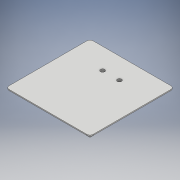
# Autodesk Inventor part: Touchplate
Saved by Autodesk Inventor 2017 (Build 210142000, 142)
## iProperties
Created: 2016-05-03
Part Number: Touchplate
Material: Generic
Document SubType Name: Modeling
Designer: alist
Density: 1 g/cm^3
Appearance: Default
Author: alist
## iProperties of the stored document Touchplate_3DPrint.ipt
Created: 2017-01-15
Part Number: Touchplate_3DPrint
Material: Generic
Document SubType Name: Modeling
Designer: Alistair
Density: 1 g/cm^3
Appearance: Default
Author: Alistair
Autodesk Inventor part; units mm, degrees
ref_plane "YZ Plane" through (0, 0, 0) normal (1, 0, 0) x (0, 1, 0)
ref_plane "XZ Plane" through (0, 0, 0) normal (0, 1, 0) x (-1, 0, 0)
ref_plane "XY Plane" through (0, 0, 0) normal (0, 0, 1) x (1, 0, 0)
sketch "Sketch1" plane through (0, 0, 0) normal (0, 0, 1) x (1, 0, 0)
  circle A0 centre (5, 0) radius 1.1 projected
  circle A1 centre (-11, 0) radius 1.1 projected
  line L0 (-11, 0) -> (5, 0) construction
  line L1 (-43, 20) -> (37, 20)
  line L2 (-3, 22.8039) -> (-3, -25.7358) construction
  line L3 (37, 20) -> (37, -60)
  line L4 (37, -60) -> (-43, -60)
  line L5 (-43, -60) -> (-43, 20)
  point P0 (0, 0)
  point P1 (-3, 0)
  point P2 (-3, 20)
  dimension "d0" = 80
  dimension "d1" = 80
  dimension "d2" = 20
  constraints: 12 end point, 2 horizontal, 2 midpoint, 2 perpendicular, 2 point on line, 2 vertical
  measures "d0" distance of L1.start L1.end
  measures "d1" distance of L1.end L3.end
  measures "d2" distance between parallel lines of L1 L0
extrude "Extrusion1" add sketch "Sketch1" along normal blind 4 contours A0 | A1 | L1 L3 L4 L5
fillet "Fillet1" radius 3 4 edges at (-43, 20, 2) (-43, -60, 2) (37, -60, 2) (37, 20, 2)
sketch "Sketch2" plane through (0, 0, 4) normal (0, 0, 1) x (1, 0, 0)
  circle A0 centre (-11, 0) radius 1.1 projected
  circle A1 centre (5, 0) radius 1.1 projected
  point P0 (0, 0)
hole "Hole1" at (-11, 0, 4) at (5, 0, 4) direction (0, 0, -1) diameter 2.1 end through all counterbore diameter 4 counterbore depth 2
chamfer "Chamfer1" distance 3 angle 45 8 edges at (-43, -20, 0) (-42.1213, 19.1213, 0) (-3, 20, 0) (36.1213, 19.1213, 0) (37, -20, 0) (36.1213, -59.1213, 0) (-3, -60, 0) (-42.1213, -59.1213, 0)
equation "\"d1\" = d0"
body "Solid1"
